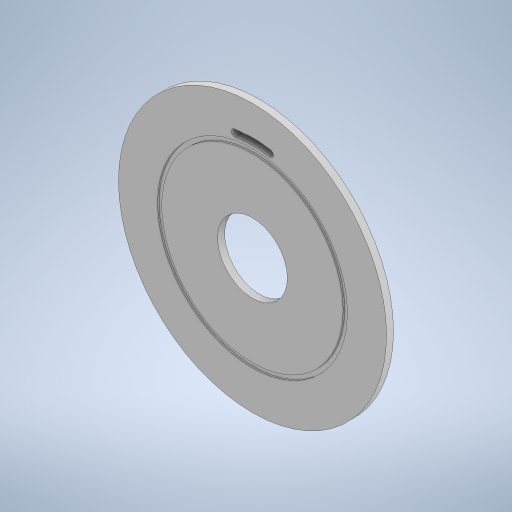
# Autodesk Inventor part: Brida_1 (flange_1)
Saved by Autodesk Inventor 2024.3 (Build 283343000, 343)
## iProperties
Created: 2025-07-02
Part Number: Brida_1 (flange_1)
Material: Genérico
Document SubType Name: Modeling
Designer: Daniel Rodriguez
Density: 1 g/cm^3
Appearance: Valor por defecto
Author: Daniel Rodriguez
Autodesk Inventor part; units mm, degrees
ref_plane "YZ Plane" through (0, 0, 0) normal (1, 0, 0) x (0, 1, 0)
ref_plane "XZ Plane" through (0, 0, 0) normal (0, 1, 0) x (-1, 0, 0)
ref_plane "XY Plane" through (0, 0, 0) normal (0, 0, 1) x (1, 0, 0)
sketch "Boceto1" plane through (0, 0, 0) normal (0, 0, 1) x (1, 0, 0)
  circle A0 centre (0, 0) radius 480
  circle A1 centre (0, 0) radius 125
  dimension "d0" = 960
  dimension "d1" = 250
  constraints: 2 centre point, 2 coincident
  measures "d0" diameter of A0
  measures "d1" diameter of A1
extrude "Extrusión1" add sketch "Boceto1" against normal blind 25
sketch "Boceto2" plane through (0, 0, 0) normal (0, 0, 1) x (1, 0, 0)
  circle A0 centre (0, 0) radius 325
  circle A1 centre (0, 0) radius 340
  dimension "d4" = 680
  dimension "d5" = 650
  constraints: 2 centre point, 2 coincident
  measures "d4" diameter of A1
  measures "d5" diameter of A0
extrude "Extrusión2" cut sketch "Boceto2" against normal blind 5
sketch "Boceto3" plane through (0, 0, 0) normal (0, 0, 1) x (1, 0, 0)
  arc A0 (63.1842, 356.4432) -> (-63.1842, 356.4432) centre (0, 0) ccw construction
  arc A1 (65.2787, 368.259) -> (-65.2787, 368.259) centre (0, 0) ccw
  arc A2 (61.0897, 344.6274) -> (-61.0897, 344.6274) centre (0, 0) ccw
  arc A3 (61.0897, 344.6274) -> (65.2787, 368.259) centre (63.1842, 356.4432) ccw
  arc A4 (-65.2787, 368.259) -> (-61.0897, 344.6274) centre (-63.1842, 356.4432) ccw
  line L0 (0, -74.8) -> (0, 448.8) projected
  point P0 (75, 354.3487)
  point P1 (-75, 354.3487)
  point P2 (0, 362)
  dimension "d8" = 12
  dimension "d9" = 362
  dimension "d15" = 150
  constraints: 13 point on circle, 5 centre point, 4 tangent, 1 coincident, 1 vertical alignment
  measures "d8" radius of A3
  measures "d9" radius of A0
  measures "d15" distance of point (75, 354.349) point (-75, 354.349)
extrude "Extrusión3" cut sketch "Boceto3" against normal up to next
